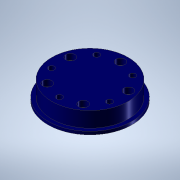
# Autodesk Inventor part: OutputShaft2
Saved by Autodesk Inventor 2021 (Build 250183000, 183)
## iProperties
Created: 2022-09-01
Part Number: OutputShaft2
Material: Ogólny
Document SubType Name: Modeling
Designer: MicnedSQ
Density: 1 g/cm^3
Appearance: Domyślna
Author: MicnedSQ
## iProperties of the stored document _Drukowanie 3D.ipt
Created: 2022-09-05
Part Number: _Drukowanie 3D
Material: Ogólny
Document SubType Name: Modeling
Designer: MicnedSQ
Density: 1 g/cm^3
Appearance: Domyślna
Author: MicnedSQ
Autodesk Inventor part; units mm, degrees
ref_plane "YZ Plane" through (0, 0, 0) normal (1, 0, 0) x (0, 1, 0)
ref_plane "XZ Plane" through (0, 0, 0) normal (0, 1, 0) x (-1, 0, 0)
ref_plane "XY Plane" through (0, 0, 0) normal (0, 0, 1) x (1, 0, 0)
sketch "Szkic4" plane through (0, 0, 0) normal (0, 1, 0) x (-1, 0, 0)
  circle A0 centre (0, 0) radius 27.5
  dimension "d13" = 55
  constraints: 1 centre point, 1 coincident
  measures "d13" diameter of A0
extrude "Wyciągnięcie proste4" add sketch "Szkic4" along normal blind 2
sketch "Szkic5" plane through (0, 2, 0) normal (0, 1, 0) x (1, 0, 0)
  circle A0 centre (0, 0) radius 25
  dimension "d16" = 50
  constraints: 1 centre point, 1 coincident
  measures "d16" diameter of A0
extrude "Wyciągnięcie proste5" add sketch "Szkic5" along normal blind 10
sketch "Szkic6" plane through (0, 12, 0) normal (0, 1, 0) x (1, 0, 0)
  circle A0 centre (0, 0) radius 20
  circle A1 centre (0, 20) radius 3
  dimension "d19" = 40
  dimension "d20" = 6
  constraints: 1 centre point, 1 coincident, 1 vertical alignment, 2 other
  measures "d20" diameter of A1
extrude "Wyciągnięcie proste6" cut sketch "Szkic6" against normal blind 4 contours A1 A0 | A0 A1 picked at (0, 18.9833) picked at (0.0861, 20.9796)
sketch "Szkic7" plane through (0, 8, -20) normal (0, 1, 0) x (1, 0, 0)
  circle A0 centre (0, 0) radius 1.65
  point P0 (0, -20)
  dimension "d23" = 3.3
  constraints: 1 centre point
  measures "d23" diameter of A0
extrude "Wyciągnięcie proste7" cut sketch "Szkic7" against normal through all
pattern_circular "Szyk kołowy2" count 5 over 360 about axis through (0, 2, 0) along (0, 1, 0) of "Wyciągnięcie proste6", "Wyciągnięcie proste7"
sketch "Szkic8" plane through (0, 12, 0) normal (0, 1, 0) x (1, 0, 0)
  circle A0 centre (0, 0) radius 20
  circle A1 centre (0, -20) radius 1.95
  dimension "d29" = 40
  dimension "d30" = 3.9
  constraints: 1 centre point, 1 coincident, 1 vertical alignment, 2 other
  measures "d30" diameter of A1
extrude "Wyciągnięcie proste8" cut sketch "Szkic8" against normal blind 8 contours A1 A0 | A0 A1 picked at (0.0759, -19.3474) picked at (0.0638, -20.6398)
pattern_circular "Szyk kołowy3" count 5 over 360 about axis through (0, 2, 0) along (0, 1, 0) of "Wyciągnięcie proste8"
